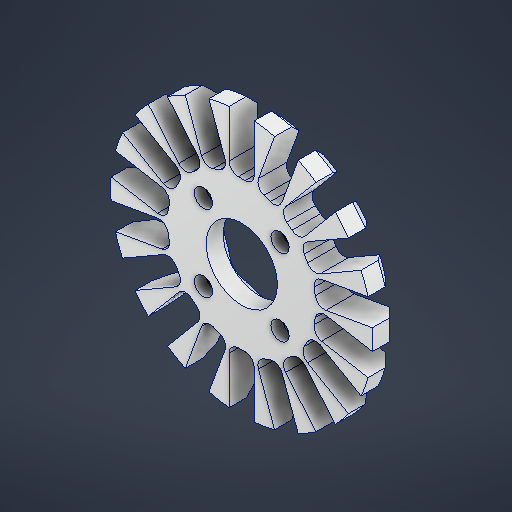
# Autodesk Inventor part: Raddeckel
Saved by Autodesk Inventor 2025.2 (Build 292293000, 293)
## iProperties
Created: 2025-03-24
Part Number: Raddeckel
Material: Generisch
Document SubType Name: Modeling
Designer: Faabs
Density: 1 g/cm^3
Appearance: Aluminium - flach
Author: Faabs
Autodesk Inventor part; units mm, degrees
ref_plane "YZ Plane" through (0, 0, 0) normal (1, 0, 0) x (0, 1, 0)
ref_plane "XZ Plane" through (0, 0, 0) normal (0, 1, 0) x (-1, 0, 0)
ref_plane "XY Plane" through (0, 0, 0) normal (0, 0, 1) x (1, 0, 0)
sketch "Skizze1" plane through (0, 0, 0) normal (0, 0, 1) x (1, 0, 0)
  line L0 (0, 0) -> (0, 5)
  line L1 (0, 0) -> (23, 0)
  line L2 (23, 0) -> (23, 3)
  line L3 (6.25, 0) -> (6.25, 5)
  line L4 (6.25, 5) -> (21, 5)
  line L5 (21, 5) -> (23, 3)
  dimension "d0" = 5
  dimension "d1" = 23
  dimension "d2" = 5
  dimension "d3" = 12.5
  dimension "d4" = 3
  dimension "d5" = 46
  dimension "d6" = 45
  constraints: 12 end point, 3 vertical, 2 horizontal, 2 point on line
  measures "d0" distance of L0.start L0.end
  measures "d1" distance of L0.start L1.end
  measures "d2" distance of L3.start L3.end
  measures "d3" diameter of L3 L0
  measures "d4" distance of L2.start L2.end
  measures "d5" diameter of L2 L0
  measures "d6" angle of L2 L5
revolve "Radkörper" add sketch "Skizze1" angle 360 about axis through (0, 0, 0) along (0, 1, 0)
sketch "Skizze2" plane through (0, 0, 0) normal (0, -1, 0) x (1, 0, 0)
  circle A0 centre (0, 0) radius 23
  circle A1 centre (0, 0) radius 13 construction
  line L0 (0, 0) -> (0, 23) construction
  line L1 (0, 23) -> (2.2, 23)
  line L2 (2.2, 23) -> (2.2, 14.6)
  line L3 (0.6, 13) -> (0, 13)
  line L4 (0, 13) -> (0, 23) construction
  line L5 (0, 23) -> (-2.2, 23)
  line L6 (-2.2, 23) -> (-2.2, 14.6)
  line L7 (-0.6, 13) -> (0, 13)
  line L8 (0, 13) -> (0, 23) construction
  arc A2 (-2.2, 14.6) -> (-0.6, 13) centre (-0.6, 14.6) ccw
  arc A3 (0.6, 13) -> (2.2, 14.6) centre (0.6, 14.6) ccw
  point P0 (2.2, 13)
  point P1 (-2.2, 13)
  point P2 (2.2, 22.8945)
  point P3 (-2.2, 22.8945)
  point P4 (0, 13)
  dimension "d8" = 46
  dimension "d9" = 26
  dimension "d10" = 2.2
  dimension "d12" = 4.4
  dimension "d15" = 1.6
  dimension "d46" = 8.4
  dimension "d47" = 8.4
  constraints: 18 end point, 4 parallel, 4 point on circle, 4 point on line, 4 tangent, 3 centre point, 2 coincident, 2 horizontal, 2 perpendicular, 1 equal radius, 1 vertical, 3 other
  measures "d9" diameter of A1
  measures "d10" distance of point (2.2, 13) L3.end
  measures "d12" distance between parallel lines of L6 L2
  measures "d15" radius of A2
  measures "d46" distance from line of L1 A3.centre
  measures "d47" distance from line of A2.centre L5
extrude "Querrolle" cut sketch "Skizze2" against normal up to surface (5 mm away) contours L2 A3 L3 L7 A2 L6 A0 picked at (0, 17.4)
pattern_circular "Runde Anordnung1" count 18 over 360 about axis through (0, -10, 0) along (0, 1, 0) of "Querrolle"
sketch "Skizze3" plane through (-2.2, 5, 20.8844) normal (0, 1, 0) x (1, 0, 0)
  circle A0 centre (2.2, 20.8844) radius 9.5 construction
  line L0 (2.2, 20.8844) -> (2.2, 11.3844) construction
  line L1 (2.2, 20.8844) -> (8.9175, 14.1669) construction
  point P0 (8.9175, 27.602)
  point P1 (-4.5175, 27.602)
  point P2 (-4.5175, 14.1669)
  dimension "d21" = 19
  dimension "d22" = 45
  dimension "d25" = 360
  constraints: 4 end point, 2 coincident, 2 point on circle, 1 centre point, 1 vertical, 5 other
  measures "d21" diameter of A0
  measures "d22" angle of L1 L0
hole "Bohrung1" at (6.7175, 5, 6.7175) at (6.7175, 5, -6.7175) at (-6.7175, 5, -6.7175) at (-6.7175, 5, 6.7175) direction (0, -1, 0) diameter 3.2 depth 5 tip angle 118 counterbore diameter 5.6 counterbore depth 3
chamfer "Fasen5" distance 2 angle 45 1 edges at (-6.25, 5, 0)
chamfer "Fasen6" distance 0.25 angle 45 6 edges at (-4.9297, 5, 8.8724) (-9.5055, 5, 6.9771) (4.9297, 5, 8.8724) (9.5055, 5, 6.9771) (-8.6974, 5, -8.6974) (8.6974, 5, -8.6974)
sketch "Skizze7" plane through (2.2, 0, 14.6) normal (0, -1, 0) x (1, 0, 0)
  circle A0 centre (-2.2, -14.6) radius 6.25
  constraints: 1 centre point, 1 coincident
extrude "Extrusion6" [suppressed]
equation "\"d1\" = 0.5 * d5"
equation "\"d2\" = d0"
